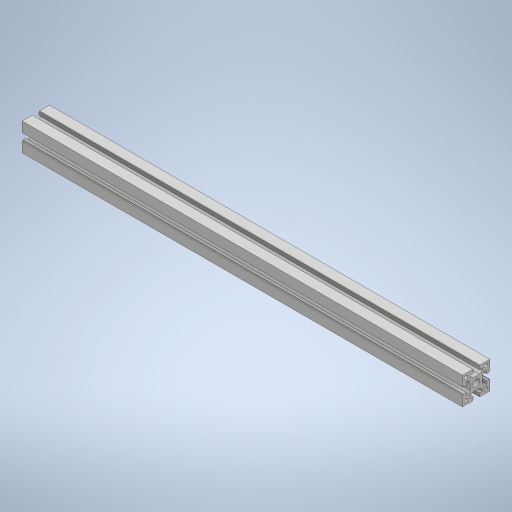
# Autodesk Inventor part: Perfil 45X45x720
Saved by Autodesk Inventor 2024.2 (Build 282272000, 272)
## iProperties
Created: 2024-05-14
Part Number: Perfil 45X45x720
Material: Genérico
Document SubType Name: Modeling
Designer: lugomez
Density: 1 g/cm^3
Appearance: Por defecto
Author: lugomez
Autodesk Inventor part; units mm, degrees
ref_plane "YZ Plane" through (0, 0, 0) normal (1, 0, 0) x (0, 1, 0)
ref_plane "XZ Plane" through (0, 0, 0) normal (0, 1, 0) x (-1, 0, 0)
ref_plane "XY Plane" through (0, 0, 0) normal (0, 0, 1) x (1, 0, 0)
sketch "Boceto1" plane through (0, 0, 0) normal (1, 0, 0) x (0, 1, 0)
  line L0 (0, 22.5) -> (16.5, 22.5)
  line L1 (16.5, 22.5) -> (16.5, 21)
  line L2 (16.5, 21) -> (17.5, 21)
  line L3 (17.5, 21) -> (17.5, 16.5)
  line L4 (17.5, 16.5) -> (12.5, 16.5)
  line L5 (12.5, 16.5) -> (12.5, 12.5)
  line L6 (12.5, 12.5) -> (17.5, 10)
  line L7 (17.5, 10) -> (27.5, 10)
  line L8 (32.5, 12.5) -> (32.5, 16.5)
  line L9 (32.5, 16.5) -> (27.5, 16.5)
  line L10 (27.5, 16.5) -> (27.5, 21)
  line L11 (27.5, 21) -> (28.5, 21)
  line L12 (28.5, 21) -> (28.5, 22.5)
  line L13 (28.5, 22.5) -> (45, 22.5)
  line L14 (45, 22.5) -> (45, 6)
  line L15 (45, 6) -> (43.5, 6)
  line L16 (43.5, 6) -> (43.5, 5)
  line L17 (43.5, 5) -> (39, 5)
  line L18 (32.5, 12.5) -> (27.5, 10)
  line L19 (0, 0) -> (0, 104.1484) construction
  line L20 (0, 0) -> (99.9828, 0) construction
  line L21 (39, 5) -> (39, 10)
  line L22 (39, 10) -> (35, 10)
  line L23 (35, 10) -> (32.5, 5)
  line L24 (32.5, 5) -> (32.5, 0)
  circle A0 centre (22.5, 0) radius 6
  circle A1 centre (39, 16.5) radius 3
  line L25 (0, 0) -> (68.012, 0) construction
  line L26 (0, -22.5) -> (16.5, -22.5)
  line L27 (16.5, -22.5) -> (16.5, -21)
  line L28 (16.5, -21) -> (17.5, -21)
  line L29 (17.5, -21) -> (17.5, -16.5)
  line L30 (17.5, -16.5) -> (12.5, -16.5)
  line L31 (12.5, -16.5) -> (12.5, -12.5)
  line L32 (12.5, -12.5) -> (17.5, -10)
  line L33 (17.5, -10) -> (27.5, -10)
  line L34 (32.5, -12.5) -> (32.5, -16.5)
  line L35 (32.5, -16.5) -> (27.5, -16.5)
  line L36 (27.5, -16.5) -> (27.5, -21)
  line L37 (27.5, -21) -> (28.5, -21)
  line L38 (28.5, -21) -> (28.5, -22.5)
  line L39 (28.5, -22.5) -> (45, -22.5)
  line L40 (45, -22.5) -> (45, -6)
  line L41 (45, -6) -> (43.5, -6)
  line L42 (43.5, -6) -> (43.5, -5)
  line L43 (43.5, -5) -> (39, -5)
  line L44 (32.5, -12.5) -> (27.5, -10)
  line L45 (39, -5) -> (39, -10)
  line L46 (39, -10) -> (35, -10)
  line L47 (35, -10) -> (32.5, -5)
  line L48 (32.5, -5) -> (32.5, 0)
  circle A2 centre (39, -16.5) radius 3
  line L49 (0, -22.5) -> (0, 22.5)
  line L50 (22.5, -24.7031) -> (22.5, 16.5) construction
  line L51 (0, 6) -> (1.5, 6)
  line L52 (1.5, 6) -> (1.5, 5)
  line L53 (1.5, 5) -> (6, 5)
  line L54 (6, 5) -> (6, 10)
  line L55 (6, 10) -> (10, 10)
  line L56 (10, 10) -> (12.5, 5)
  line L57 (12.5, 5) -> (12.5, 0)
  line L58 (1.5, -6) -> (1.5, -5)
  line L59 (0, -6) -> (1.5, -6)
  line L60 (10, -10) -> (12.5, -5)
  line L61 (6, -5) -> (6, -10)
  line L62 (6, -10) -> (10, -10)
  line L63 (1.5, -5) -> (6, -5)
  line L64 (12.5, -5) -> (12.5, 0)
  circle A3 centre (6, 16.5) radius 3
  circle A4 centre (6, -16.5) radius 3
  point P0 (22.5, 10)
  point P1 (22.5, -10)
  dimension "d1" = 22.5
  dimension "d3" = 20
  dimension "d4" = 1.5
  dimension "d5" = 1.5
  dimension "d6" = 10
  dimension "d7" = 12
  dimension "d8" = 12.5
  dimension "d9" = 22.5
  dimension "d10" = 5
  dimension "d11" = 6
  dimension "d12" = 10
  dimension "d13" = 6
  dimension "d14" = 4
  dimension "d15" = 5
  dimension "d17" = 6
  dimension "d18" = 45
  dimension "d20" = 10
  dimension "d21" = 4
  dimension "d22" = 12.5
  dimension "d23" = 6
  dimension "d24" = 12
  dimension "d25" = 22.5
  dimension "d26" = 6
  dimension "d27" = 39
  dimension "d28" = 16.5
  dimension "d31" = 12.5
  constraints: 130 end point, 42 symmetric about line, 13 point on line, 12 perpendicular, 5 centre point, 4 vertical, 3 horizontal alignment, 2 coincident, 2 collinear, 2 horizontal, 2 midpoint, 2 parallel, 1 vertical alignment, 3 other
  measures "d1" distance from line of point (0, 0) L0
  measures "d3" distance between parallel lines of L5 L8
  measures "d4" distance between parallel lines of L0 L2
  measures "d5" distance between parallel lines of L14 L16
  measures "d6" distance between parallel lines of L10 L3
  measures "d7" distance between parallel lines of L1 L12
  measures "d8" distance between parallel lines of L0 L7
  measures "d9" horizontal distance of point (22.5, 10) point (0, 0)
  measures "d10" distance from line of point (22.5, 10) L10
  measures "d11" distance from line of point (22.5, 10) L12
  measures "d12" distance from line of point (22.5, 10) L5
  measures "d13" distance between parallel lines of L0 L4
  measures "d14" distance of L4.end L5.end
  measures "d15" distance between parallel lines of L20 L17
  measures "d17" distance between parallel lines of L20 L15
  measures "d18" distance from line of point (0, 0) L14
  measures "d20" distance between parallel lines of L20 L22
  measures "d21" distance of L21.end L22.end
  measures "d22" distance between parallel lines of L14 L24
  measures "d23" distance between parallel lines of L14 L21
  measures "d24" diameter of A0
  measures "d25" distance of point (0, 0) A0.centre
  measures "d26" diameter of A1
  measures "d27" horizontal distance of A1.centre point (0, 0)
  measures "d28" vertical distance of point (0, 0) A1.centre
  measures "d31" distance from line of point (0, 0) L57
extrude "Perfil base" add sketch "Boceto1" along normal blind 720 contours L0 L1 L2 L3 L4 L5 L6 L7 L18 L8 L9 L10 L11 L12 L13 L14 L15 L16 L17 L21 L22 L23 L24 L48 L47 L46 L45 L43 L42 L41 L40 L39 L38 L37 L36 L35 L34 L44 L33 L32 L31 L30 L29 L28 L27 L26 L49 L59 L58 L63 L61 L62 L60 L64 L57 L56 L55 L54 L53 L52 L51
equation "\"d5\" = d4"
equation "\"d10\" = 0.5 * d6"
equation "\"d11\" = 0.5 * d7"
equation "\"d12\" = 0.5 * d3"
equation "\"d15\" = d10"
equation "\"d17\" = d11"
equation "\"d20\" = d12"
equation "\"d21\" = d14"
equation "\"d23\" = d13"
